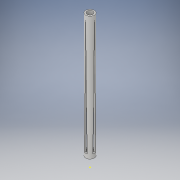
# Autodesk Inventor part: steam pipe
Saved by Autodesk Inventor 2019 (Build 230136000, 136)
## iProperties
Created: 2019-06-12
Part Number: steam pipe
Material: Generic
Document SubType Name: Modeling
Designer: Admin
Density: 1 g/cm^3
Appearance: Default
Author: Admin
Autodesk Inventor part; units mm, degrees
ref_plane "XZ Plane" through (0, 0, 0) normal (0, 1, 0) x (-1, 0, 0)
sketch "Sketch1" plane through (0, 0, 0) normal (0, 1, 0) x (-1, 0, 0)
  circle A0 centre (0, 0) radius 15
  dimension "d0" = 30
  constraints: 1 centre point, 1 coincident
  measures "d0" diameter of A0
extrude "Extrusion1" add sketch "Sketch1" along normal blind 500
ref_plane "Work Plane1" through (15, 0, 0) normal (1, 0, 0) x (0, 1, 0)
sketch "Sketch2" plane through (15, 0, 0) normal (1, 0, 0) x (0, 1, 0)
  line L0 (50, 4.712) -> (50, -4.713)
  line L1 (450, 0) -> (50, -4.713)
  line L2 (50, 4.712) -> (450, 0)
  point P0 (0, 0)
  dimension "d4" = 9.425
  constraints: 6 end point, 1 vertical
  measures "d4" distance of L0.start L0.end
extrude "Extrusion2" cut sketch "Sketch2" against normal blind 500
ref_plane "Work Plane2" through (0, 0, 15) normal (0, 0, 1) x (1, 0, 0)
sketch "Sketch3" plane through (0, 0, 15) normal (0, 0, 1) x (1, 0, 0)
  line L0 (4.712, 50) -> (-4.713, 50)
  line L1 (0, 450) -> (4.712, 50)
  line L2 (0, 450) -> (-4.713, 50)
  point P0 (0, 0)
  dimension "d8" = 9.425
  constraints: 6 end point
  measures "d8" distance of L0.start L0.end
extrude "Extrusion3" cut sketch "Sketch3" against normal blind 500
sketch "Sketch4" plane through (0, 500, 0) normal (0, 1, 0) x (1, 0, 0)
  circle A0 centre (0, 0) radius 10
  dimension "d11" = 20
  constraints: 1 centre point, 1 coincident
  measures "d11" diameter of A0
extrude "Extrusion4" cut sketch "Sketch4" against normal blind 500
sketch "Sketch5" plane through (0, 500, 0) normal (0, 1, 0) x (1, 0, 0)
  circle A0 centre (0, 0) radius 15
  constraints: 1 centre point, 1 coincident
extrude "Extrusion5" cut sketch "Sketch5" against normal blind 10
sketch "Sketch6" plane through (0, 0, 0) normal (0, -1, 0) x (1, 0, 0)
  circle A0 centre (0, 0) radius 15
  constraints: 1 centre point, 1 coincident
extrude "Extrusion6" cut sketch "Sketch6" against normal blind 10
sketch "Sketch7" plane through (0, 0, 0) normal (0, 0, 1) x (1, 0, 0)
  point P0 (0, 0)
sketch "Sketch8" plane through (0, 10, 0) normal (0, -1, 0) x (1, 0, 0)
  circle A0 centre (0, 0) radius 15
  constraints: 1 centre point, 1 coincident
extrude "Extrusion7" cut sketch "Sketch8" against normal blind 10
sketch "Sketch9" plane through (0, 490, 0) normal (0, 1, 0) x (1, 0, 0)
  circle A0 centre (0, 0) radius 10 projected
  circle A1 centre (0, 0) radius 15
  constraints: 1 centre point, 1 coincident
extrude "Extrusion8" cut sketch "Sketch9" against normal blind 10
sketch "Sketch10" plane through (0, 20, 0) normal (0, -1, 0) x (1, 0, 0)
  arc A0 (14.2404, -4.713) -> (14.2407, 4.712) centre (0, 0) ccw projected
  circle A1 centre (0, 0) radius 15
  constraints: 1 coincident, 3 other
extrude "Extrusion9" cut sketch "Sketch10" against normal blind 15
sketch "Sketch11" plane through (0, 480, 0) normal (0, 1, 0) x (1, 0, 0)
  arc A0 (14.2407, -4.712) -> (15, 0) centre (0, 0) ccw projected
  circle A1 centre (0, 0) radius 15
  constraints: 1 coincident, 1 horizontal alignment, 2 other
extrude "Extrusion10" cut sketch "Sketch11" against normal blind 15
body "Solid1"
